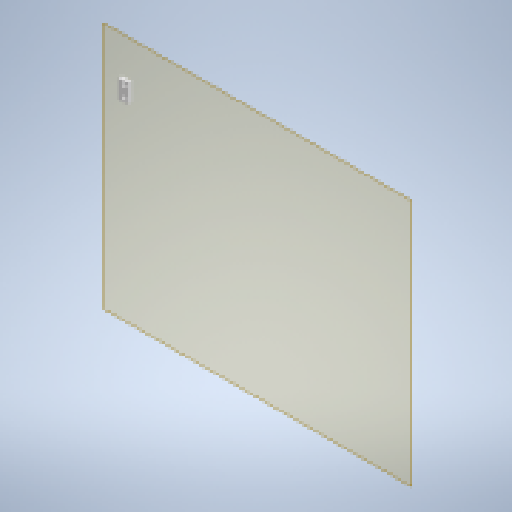
# Autodesk Inventor part: soporte pantalla 2
Saved by Autodesk Inventor 2023 (Build 270158000, 158)
## iProperties
Created: 2023-05-20
Part Number: soporte pantalla 2
Material: Genérico
Document SubType Name: Modeling
Designer: sergi
Density: 1 g/cm^3
Appearance: Valor por defecto
Author: sergi
Autodesk Inventor part; units mm, degrees
ref_plane "YZ Plane" through (0, 0, 0) normal (1, 0, 0) x (0, 1, 0)
ref_plane "XZ Plane" through (0, 0, 0) normal (0, 1, 0) x (-1, 0, 0)
ref_plane "XY Plane" through (0, 0, 0) normal (0, 0, 1) x (1, 0, 0)
ref_plane "Plano de trabajo1" through (0, 0, 0) normal (0, 0, 1) x (1, 0, 0)
sketch "Boceto1" plane through (0, 0, 0) normal (0, 0, 1) x (1, 0, 0)
  circle A0 centre (36.5, 9) radius 1.5 projected
  circle A1 centre (-11.85, 9) radius 1.5 projected
  circle A2 centre (84.85, 9) radius 1.5 projected
  line L0 (-112.15, 0) -> (105.85, 0) projected
  line L1 (105.85, 0) -> (105.85, 146.9) projected
  line L2 (105.85, 146.9) -> (112.15, 146.9) projected
  line L3 (112.15, 146.9) -> (112.15, 160) projected
  line L4 (112.15, 160) -> (105.85, 160) projected
  line L5 (105.85, 160) -> (105.85, 180) projected
  line L6 (105.85, 180) -> (-100.9, 180) projected
  line L7 (-100.9, 180) -> (-100.9, 160) projected
  line L8 (-100.9, 160) -> (-108.4, 160) projected
  line L9 (-108.4, 160) -> (-108.4, 145) projected
  line L10 (-108.4, 145) -> (-100.9, 145) projected
  line L11 (-100.9, 145) -> (-100.9, 142) projected
  line L12 (-100.9, 142) -> (-112.15, 142) projected
  line L13 (-112.15, 142) -> (-112.15, 0) projected
  circle A3 centre (108.75, 156.3) radius 1.5 projected
  circle A4 centre (-103.8, 148.3) radius 1.5 projected
  circle A5 centre (-103.8, 156.7) radius 1.5 projected
  circle A6 centre (108.75, 150.6) radius 1.5 projected
  line L14 (-14.65, 175.8) -> (-14.65, 157.7) projected
  line L15 (-14.65, 157.7) -> (-22.65, 157.7) projected
  line L16 (-22.65, 157.7) -> (-22.65, 175.8) projected
  line L17 (-22.65, 175.8) -> (-14.65, 175.8) projected
  line L18 (56.65, 169.8) -> (56.65, 163.3) projected
  line L19 (56.65, 163.3) -> (50.15, 163.3) projected
  line L20 (50.15, 163.3) -> (50.15, 169.8) projected
  line L21 (50.15, 169.8) -> (56.65, 169.8) projected
  line L22 (38.55, 169.8) -> (38.55, 163.3) projected
  line L23 (38.55, 163.3) -> (32.05, 163.3) projected
  line L24 (32.05, 163.3) -> (32.05, 169.8) projected
  line L25 (32.05, 169.8) -> (38.55, 169.8) projected
  line L26 (-4.15, 163.3) -> (-4.15, 169.8) projected
  line L27 (-4.15, 169.8) -> (2.35, 169.8) projected
  line L28 (2.35, 169.8) -> (2.35, 163.3) projected
  line L29 (2.35, 163.3) -> (-4.15, 163.3) projected
  line L30 (78.15, 169.8) -> (78.15, 163.3) projected
  line L31 (78.15, 163.3) -> (71.65, 163.3) projected
  line L32 (71.65, 163.3) -> (71.65, 169.8) projected
  line L33 (71.65, 169.8) -> (78.15, 169.8) projected
  line L34 (20.45, 169.8) -> (20.45, 163.3) projected
  line L35 (20.45, 163.3) -> (13.95, 163.3) projected
  line L36 (13.95, 163.3) -> (13.95, 169.8) projected
  line L37 (13.95, 169.8) -> (20.45, 169.8) projected
  circle A7 centre (-62.15, 35) radius 1.6 projected
  circle A8 centre (-37.15, 35) radius 1.6 projected
  line L38 (-85.9, 15) -> (-97.15, 15) projected
  line L39 (-97.15, 15) -> (-97.15, 127) projected
  line L40 (-97.15, 127) -> (-85.9, 127) projected
  line L41 (-85.9, 127) -> (-85.9, 165) projected
  line L42 (-85.9, 165) -> (-57.05, 165) projected
  line L43 (-57.05, 165) -> (-57.05, 48.4) projected
  line L44 (-57.05, 48.4) -> (-85.9, 48.4) projected
  line L45 (-85.9, 48.4) -> (-85.9, 15) projected
  line L46 (-17.85, 15) -> (-17.85, 150.7) projected
  line L47 (-17.85, 150.7) -> (90.85, 150.7) projected
  line L48 (90.85, 150.7) -> (90.85, 15) projected
  line L49 (90.85, 15) -> (-17.85, 15) projected
  line L50 (-100.9, 145) -> (-100.9, 160)
  point P0 (0, 0)
  constraints: 2 end point, 1 vertical
extrude "Extrusión1" add sketch "Boceto1" along normal blind 3 contours L10 L9 L8 L50
